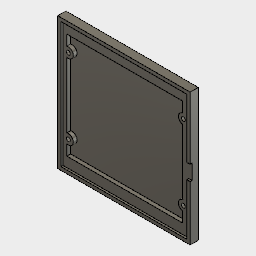
lpcCNC_Base v7 (Autodesk Fusion 360 design; units mm, degrees)
Autodesk Fusion 360 part; units mm, degrees
note: some values were not read from the file. Set by a fixed rule: which sketch regions a step uses.
sketch "Sketch1" plane through (0, 0, 0) normal (0, 0, 1) x (1, 0, 0)
  line L0 (0, 0) -> (106, 0)
  line L1 (106, 0) -> (106, 106)
  line L2 (106, 106) -> (0, 106)
  line L3 (0, 106) -> (0, 0)
  line L4 (2.75, 2.75) -> (103.25, 2.75)
  line L5 (103.25, 2.75) -> (103.25, 103.25)
  line L6 (103.25, 103.25) -> (2.75, 103.25)
  line L7 (2.75, 103.25) -> (2.75, 2.75)
  circle A0 centre (7, 23) radius 4
  circle A1 centre (7, 83) radius 4
  circle A2 centre (99, 23) radius 4
  circle A3 centre (99, 83) radius 4
  line L8 (2.75, 103.25) -> (103.25, 103.25)
  line L9 (103.25, 103.25) -> (103.25, 95.25)
  line L10 (103.25, 95.25) -> (2.75, 95.25)
  line L11 (2.75, 95.25) -> (2.75, 103.25)
  line L12 (2.75, 2.75) -> (103.25, 2.75)
  line L13 (103.25, 2.75) -> (103.25, 10.75)
  line L14 (103.25, 10.75) -> (2.75, 10.75)
  line L15 (2.75, 10.75) -> (2.75, 2.75)
  line L16 (2.75, 95.25) -> (5.75, 95.25)
  line L17 (5.75, 95.25) -> (5.75, 10.75)
  line L18 (5.75, 10.75) -> (2.75, 10.75)
  line L19 (2.75, 10.75) -> (2.75, 95.25)
  line L20 (103.25, 95.25) -> (98.25, 95.25)
  line L21 (98.25, 95.25) -> (98.25, 10.75)
  line L22 (98.25, 10.75) -> (103.25, 10.75)
  line L23 (103.25, 10.75) -> (103.25, 95.25)
  circle A4 centre (7, 83) radius 1.55
  circle A5 centre (99, 83) radius 1.55
  circle A6 centre (7, 23) radius 1.55
  circle A7 centre (99, 23) radius 1.55
  line L24 (103.25, 56) -> (106, 56)
  line L25 (106, 56) -> (106, 44)
  line L26 (106, 44) -> (103.25, 44)
  line L27 (103.25, 44) -> (103.25, 56)
  dimension "d1" = 106
  dimension "d2" = 106
  dimension "d3" = 100.5
  dimension "d4" = 100.5
  dimension "d5" = 2.75
  dimension "d6" = 2.75
  dimension "d7" = 8
  dimension "d8" = 8
  dimension "d9" = 8
  dimension "d10" = 8
  dimension "d12" = 7
  dimension "d13" = 7
  dimension "d16" = 7
  dimension "d17" = 7
  dimension "d18" = 8
  dimension "d19" = 8
  dimension "d20" = 5
  dimension "d21" = 3
  dimension "d22" = 3.1
  dimension "d23" = 3.1
  dimension "d24" = 3.1
  dimension "d25" = 3.1
  dimension "d48" = 23
  dimension "d49" = 23
  dimension "d50" = 23
  dimension "d51" = 23
  dimension "d52" = 12
  dimension "d55" = 41.25
  measures "d1" distance of L0.start L0.end
  measures "d2" distance of L0.start L2.end
  measures "d3" distance of L4.start L4.end
  measures "d4" distance of L4.start L6.end
  measures "d5" distance of L3 L7
  measures "d6" distance of L2 L6
  measures "d7" diameter of A0
  measures "d8" diameter of A1
  measures "d9" diameter of A2
  measures "d10" diameter of A3
  measures "d12" distance of L3 A0.centre
  measures "d13" distance of L3 A1.centre
  measures "d16" distance of L1 A3.centre
  measures "d17" distance of L1 A2.centre
  measures "d18" distance of L6 L10
  measures "d19" distance of L12 L14
  measures "d20" distance of L5 L21
  measures "d21" distance of L17 L19
  measures "d22" diameter of A4
  measures "d23" diameter of A5
  measures "d24" diameter of A6
  measures "d25" diameter of A7
  measures "d48" distance of L2 A1.centre
  measures "d49" distance of L2 A3.centre
  measures "d50" distance of L0 A0.centre
  measures "d51" distance of L0 A2.centre
  measures "d52" distance of L24 L26
  measures "d55" distance of L12 L26
extrude "Extrude1" add sketch "Sketch1" against normal blind 2 contours L0 L1 L2 L3 L4 L5 L6 L7 L8 L9 L11 L12 L13 L15 L19 L23 L24 L26 | L1 L5 L23 L24 L25 L26 L27 | L5 A2 A3 L10 L14 L20 L21 L22 L23 L27 | L4 L5 L7 L12 L13 L14 L15 L18 L22 | L5 L6 L7 L8 L9 L10 L11 L16 L20 | A0 A1 A2 A3 L10 L14 L17 L21 | L7 A0 A1 L10 L14 L16 L17 L18 L19 | A2 L21 A7 | A2 L21 A7 | A3 L21 A5 | A3 L21 A5 | A0 L17 A6 | A0 L17 A6 | A1 L17 A4 | A1 L17 A4
extrude "Extrude2" add sketch "Sketch1" along normal blind 4.6 contours L0 L1 L2 L3 L4 L5 L6 L7 L8 L9 L11 L12 L13 L15 L19 L23 L24 L26
extrude "Extrude3" add sketch "Sketch1" along normal blind 3 contours L1 L5 L23 L24 L25 L26 L27 | L5 A2 A3 L10 L14 L20 L21 L22 L23 L27 | L4 L5 L7 L12 L13 L14 L15 L18 L22 | L5 L6 L7 L8 L9 L10 L11 L16 L20 | L7 A0 A1 L10 L14 L16 L17 L18 L19 | A2 L21 A7 | A2 L21 A7 | A3 L21 A5 | A3 L21 A5 | A0 L17 A6 | A0 L17 A6 | A1 L17 A4 | A1 L17 A4
